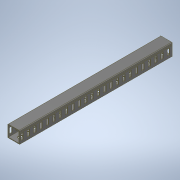
# Autodesk Inventor part: 503.009.01_Kabelkanal
Saved by Autodesk Inventor 2021 (Build 250183000, 183)
## iProperties
Created: 2021-11-27
Part Number: 503.009.01_Kabelkanal
Material: Polypropylen
Document SubType Name: Modeling
Designer: Sebastian Seewald
Density: 0.899 g/cm^3
Appearance: Glatt - Esche
Mass: 114.345 g
Surface Area: 1336.96 cm^2
Volume: 127.191 cm^3
Author: Sebastian Seewald
Autodesk Inventor part; units mm, degrees
ref_plane "YZ Plane" through (0, 0, 0) normal (1, 0, 0) x (0, 1, 0)
ref_plane "XZ Plane" through (0, 0, 0) normal (0, 1, 0) x (-1, 0, 0)
sketch "Skizze1" plane through (0, 0, 0) normal (0, 0, 1) x (1, 0, 0)
  line L0 (0, 0) -> (37.5, 0)
  line L1 (37.5, 0) -> (37.5, 35.5)
  line L2 (35.5, 37.5) -> (2, 37.5)
  line L3 (0, 35.5) -> (0, 0)
  line L4 (4, 35.5) -> (33.5, 35.5)
  line L5 (35.5, 33.5) -> (35.5, 2)
  line L6 (35.5, 2) -> (2, 2)
  line L7 (2, 2) -> (2, 33.5)
  arc A0 (2, 37.5) -> (0, 35.5) centre (2, 35.5) ccw
  arc A1 (37.5, 35.5) -> (35.5, 37.5) centre (35.5, 35.5) ccw
  arc A2 (35.5, 33.5) -> (33.5, 35.5) centre (33.5, 33.5) ccw
  arc A3 (4, 35.5) -> (2, 33.5) centre (4, 33.5) ccw
  point P0 (37.5, 37.5)
  point P1 (0, 37.5)
  dimension "d0" = 37.5
  dimension "d1" = 37.5
  dimension "d2" = 2
  dimension "d3" = 2
  dimension "d4" = 2
  dimension "d5" = 2
  dimension "d6" = 2
  constraints: 16 end point, 8 point on circle, 8 tangent, 4 centre point, 4 parallel, 4 point on line, 3 equal radius, 2 horizontal, 2 perpendicular
  measures "d0" distance of point (37.5, 37.5) point (0, 37.5)
  measures "d1" distance of L0.end point (37.5, 37.5)
  measures "d2" distance between parallel lines of L3 L7
  measures "d3" distance between parallel lines of L2 L4
  measures "d4" distance between parallel lines of L1 L5
  measures "d5" distance between parallel lines of L0 L6
  measures "d6" radius of A0
extrude "Extrusion1" add sketch "Skizze1" along normal blind 480
sketch "Skizze2" plane through (0, 0, 0) normal (-1, 0, 0) x (0, 0, 1)
  line L0 (9, 26.5) -> (15, 26.5)
  line L1 (16, 25.5) -> (16, 9)
  line L2 (15, 8) -> (9, 8)
  line L3 (8, 9) -> (8, 25.5)
  line L4 (0, 0) -> (480, 0) projected
  line L5 (0, 35.5) -> (0, 0) projected
  arc A0 (9, 26.5) -> (8, 25.5) centre (9, 25.5) ccw
  arc A1 (16, 25.5) -> (15, 26.5) centre (15, 25.5) ccw
  arc A2 (15, 8) -> (16, 9) centre (15, 9) ccw
  arc A3 (8, 9) -> (9, 8) centre (9, 9) ccw
  line L6 (29, 26.5) -> (35, 26.5)
  line L7 (36, 25.5) -> (36, 9)
  line L8 (35, 8) -> (29, 8)
  line L9 (28, 9) -> (28, 25.5)
  arc A4 (29, 26.5) -> (28, 25.5) centre (29, 25.5) ccw
  arc A5 (36, 25.5) -> (35, 26.5) centre (35, 25.5) ccw
  arc A6 (35, 8) -> (36, 9) centre (35, 9) ccw
  arc A7 (28, 9) -> (29, 8) centre (29, 9) ccw
  line L10 (49, 26.5) -> (55, 26.5)
  line L11 (56, 25.5) -> (56, 9)
  line L12 (55, 8) -> (49, 8)
  line L13 (48, 9) -> (48, 25.5)
  arc A8 (49, 26.5) -> (48, 25.5) centre (49, 25.5) ccw
  arc A9 (56, 25.5) -> (55, 26.5) centre (55, 25.5) ccw
  arc A10 (55, 8) -> (56, 9) centre (55, 9) ccw
  arc A11 (48, 9) -> (49, 8) centre (49, 9) ccw
  line L14 (69, 26.5) -> (75, 26.5)
  line L15 (76, 25.5) -> (76, 9)
  line L16 (75, 8) -> (69, 8)
  line L17 (68, 9) -> (68, 25.5)
  arc A12 (69, 26.5) -> (68, 25.5) centre (69, 25.5) ccw
  arc A13 (76, 25.5) -> (75, 26.5) centre (75, 25.5) ccw
  arc A14 (75, 8) -> (76, 9) centre (75, 9) ccw
  arc A15 (68, 9) -> (69, 8) centre (69, 9) ccw
  line L18 (89, 26.5) -> (95, 26.5)
  line L19 (96, 25.5) -> (96, 9)
  line L20 (95, 8) -> (89, 8)
  line L21 (88, 9) -> (88, 25.5)
  arc A16 (89, 26.5) -> (88, 25.5) centre (89, 25.5) ccw
  arc A17 (96, 25.5) -> (95, 26.5) centre (95, 25.5) ccw
  arc A18 (95, 8) -> (96, 9) centre (95, 9) ccw
  arc A19 (88, 9) -> (89, 8) centre (89, 9) ccw
  line L22 (109, 26.5) -> (115, 26.5)
  line L23 (116, 25.5) -> (116, 9)
  line L24 (115, 8) -> (109, 8)
  line L25 (108, 9) -> (108, 25.5)
  arc A20 (109, 26.5) -> (108, 25.5) centre (109, 25.5) ccw
  arc A21 (116, 25.5) -> (115, 26.5) centre (115, 25.5) ccw
  arc A22 (115, 8) -> (116, 9) centre (115, 9) ccw
  arc A23 (108, 9) -> (109, 8) centre (109, 9) ccw
  line L26 (129, 26.5) -> (135, 26.5)
  line L27 (136, 25.5) -> (136, 9)
  line L28 (135, 8) -> (129, 8)
  line L29 (128, 9) -> (128, 25.5)
  arc A24 (129, 26.5) -> (128, 25.5) centre (129, 25.5) ccw
  arc A25 (136, 25.5) -> (135, 26.5) centre (135, 25.5) ccw
  arc A26 (135, 8) -> (136, 9) centre (135, 9) ccw
  arc A27 (128, 9) -> (129, 8) centre (129, 9) ccw
  line L30 (149, 26.5) -> (155, 26.5)
  line L31 (156, 25.5) -> (156, 9)
  line L32 (155, 8) -> (149, 8)
  line L33 (148, 9) -> (148, 25.5)
  arc A28 (149, 26.5) -> (148, 25.5) centre (149, 25.5) ccw
  arc A29 (156, 25.5) -> (155, 26.5) centre (155, 25.5) ccw
  arc A30 (155, 8) -> (156, 9) centre (155, 9) ccw
  arc A31 (148, 9) -> (149, 8) centre (149, 9) ccw
  line L34 (169, 26.5) -> (175, 26.5)
  line L35 (176, 25.5) -> (176, 9)
  line L36 (175, 8) -> (169, 8)
  line L37 (168, 9) -> (168, 25.5)
  arc A32 (169, 26.5) -> (168, 25.5) centre (169, 25.5) ccw
  arc A33 (176, 25.5) -> (175, 26.5) centre (175, 25.5) ccw
  arc A34 (175, 8) -> (176, 9) centre (175, 9) ccw
  arc A35 (168, 9) -> (169, 8) centre (169, 9) ccw
  line L38 (189, 26.5) -> (195, 26.5)
  line L39 (196, 25.5) -> (196, 9)
  line L40 (195, 8) -> (189, 8)
  line L41 (188, 9) -> (188, 25.5)
  arc A36 (189, 26.5) -> (188, 25.5) centre (189, 25.5) ccw
  arc A37 (196, 25.5) -> (195, 26.5) centre (195, 25.5) ccw
  arc A38 (195, 8) -> (196, 9) centre (195, 9) ccw
  arc A39 (188, 9) -> (189, 8) centre (189, 9) ccw
  line L42 (209, 26.5) -> (215, 26.5)
  line L43 (216, 25.5) -> (216, 9)
  line L44 (215, 8) -> (209, 8)
  line L45 (208, 9) -> (208, 25.5)
  arc A40 (209, 26.5) -> (208, 25.5) centre (209, 25.5) ccw
  arc A41 (216, 25.5) -> (215, 26.5) centre (215, 25.5) ccw
  arc A42 (215, 8) -> (216, 9) centre (215, 9) ccw
  arc A43 (208, 9) -> (209, 8) centre (209, 9) ccw
  line L46 (229, 26.5) -> (235, 26.5)
  line L47 (236, 25.5) -> (236, 9)
  line L48 (235, 8) -> (229, 8)
  line L49 (228, 9) -> (228, 25.5)
  arc A44 (229, 26.5) -> (228, 25.5) centre (229, 25.5) ccw
  arc A45 (236, 25.5) -> (235, 26.5) centre (235, 25.5) ccw
  arc A46 (235, 8) -> (236, 9) centre (235, 9) ccw
  arc A47 (228, 9) -> (229, 8) centre (229, 9) ccw
  line L50 (249, 26.5) -> (255, 26.5)
  line L51 (256, 25.5) -> (256, 9)
  line L52 (255, 8) -> (249, 8)
  line L53 (248, 9) -> (248, 25.5)
  arc A48 (249, 26.5) -> (248, 25.5) centre (249, 25.5) ccw
  arc A49 (256, 25.5) -> (255, 26.5) centre (255, 25.5) ccw
  arc A50 (255, 8) -> (256, 9) centre (255, 9) ccw
  arc A51 (248, 9) -> (249, 8) centre (249, 9) ccw
  line L54 (269, 26.5) -> (275, 26.5)
  line L55 (276, 25.5) -> (276, 9)
  line L56 (275, 8) -> (269, 8)
  line L57 (268, 9) -> (268, 25.5)
  arc A52 (269, 26.5) -> (268, 25.5) centre (269, 25.5) ccw
  arc A53 (276, 25.5) -> (275, 26.5) centre (275, 25.5) ccw
  arc A54 (275, 8) -> (276, 9) centre (275, 9) ccw
  arc A55 (268, 9) -> (269, 8) centre (269, 9) ccw
  line L58 (289, 26.5) -> (295, 26.5)
  line L59 (296, 25.5) -> (296, 9)
  line L60 (295, 8) -> (289, 8)
  line L61 (288, 9) -> (288, 25.5)
  arc A56 (289, 26.5) -> (288, 25.5) centre (289, 25.5) ccw
  arc A57 (296, 25.5) -> (295, 26.5) centre (295, 25.5) ccw
  arc A58 (295, 8) -> (296, 9) centre (295, 9) ccw
  arc A59 (288, 9) -> (289, 8) centre (289, 9) ccw
  line L62 (309, 26.5) -> (315, 26.5)
  line L63 (316, 25.5) -> (316, 9)
  line L64 (315, 8) -> (309, 8)
  line L65 (308, 9) -> (308, 25.5)
  arc A60 (309, 26.5) -> (308, 25.5) centre (309, 25.5) ccw
  arc A61 (316, 25.5) -> (315, 26.5) centre (315, 25.5) ccw
  arc A62 (315, 8) -> (316, 9) centre (315, 9) ccw
  arc A63 (308, 9) -> (309, 8) centre (309, 9) ccw
  line L66 (329, 26.5) -> (335, 26.5)
  line L67 (336, 25.5) -> (336, 9)
  line L68 (335, 8) -> (329, 8)
  line L69 (328, 9) -> (328, 25.5)
  arc A64 (329, 26.5) -> (328, 25.5) centre (329, 25.5) ccw
  arc A65 (336, 25.5) -> (335, 26.5) centre (335, 25.5) ccw
  arc A66 (335, 8) -> (336, 9) centre (335, 9) ccw
  arc A67 (328, 9) -> (329, 8) centre (329, 9) ccw
  line L70 (349, 26.5) -> (355, 26.5)
  line L71 (356, 25.5) -> (356, 9)
  line L72 (355, 8) -> (349, 8)
  line L73 (348, 9) -> (348, 25.5)
  arc A68 (349, 26.5) -> (348, 25.5) centre (349, 25.5) ccw
  arc A69 (356, 25.5) -> (355, 26.5) centre (355, 25.5) ccw
  arc A70 (355, 8) -> (356, 9) centre (355, 9) ccw
  arc A71 (348, 9) -> (349, 8) centre (349, 9) ccw
  line L74 (369, 26.5) -> (375, 26.5)
  line L75 (376, 25.5) -> (376, 9)
  line L76 (375, 8) -> (369, 8)
  line L77 (368, 9) -> (368, 25.5)
  arc A72 (369, 26.5) -> (368, 25.5) centre (369, 25.5) ccw
  arc A73 (376, 25.5) -> (375, 26.5) centre (375, 25.5) ccw
  arc A74 (375, 8) -> (376, 9) centre (375, 9) ccw
  arc A75 (368, 9) -> (369, 8) centre (369, 9) ccw
  line L78 (389, 26.5) -> (395, 26.5)
  line L79 (396, 25.5) -> (396, 9)
  line L80 (395, 8) -> (389, 8)
  line L81 (388, 9) -> (388, 25.5)
  arc A76 (389, 26.5) -> (388, 25.5) centre (389, 25.5) ccw
  arc A77 (396, 25.5) -> (395, 26.5) centre (395, 25.5) ccw
  arc A78 (395, 8) -> (396, 9) centre (395, 9) ccw
  arc A79 (388, 9) -> (389, 8) centre (389, 9) ccw
  line L82 (409, 26.5) -> (415, 26.5)
  line L83 (416, 25.5) -> (416, 9)
  line L84 (415, 8) -> (409, 8)
  line L85 (408, 9) -> (408, 25.5)
  arc A80 (409, 26.5) -> (408, 25.5) centre (409, 25.5) ccw
  arc A81 (416, 25.5) -> (415, 26.5) centre (415, 25.5) ccw
  arc A82 (415, 8) -> (416, 9) centre (415, 9) ccw
  arc A83 (408, 9) -> (409, 8) centre (409, 9) ccw
  line L86 (429, 26.5) -> (435, 26.5)
  line L87 (436, 25.5) -> (436, 9)
  line L88 (435, 8) -> (429, 8)
  line L89 (428, 9) -> (428, 25.5)
  arc A84 (429, 26.5) -> (428, 25.5) centre (429, 25.5) ccw
  arc A85 (436, 25.5) -> (435, 26.5) centre (435, 25.5) ccw
  arc A86 (435, 8) -> (436, 9) centre (435, 9) ccw
  arc A87 (428, 9) -> (429, 8) centre (429, 9) ccw
  line L90 (449, 26.5) -> (455, 26.5)
  line L91 (456, 25.5) -> (456, 9)
  line L92 (455, 8) -> (449, 8)
  line L93 (448, 9) -> (448, 25.5)
  arc A88 (449, 26.5) -> (448, 25.5) centre (449, 25.5) ccw
  arc A89 (456, 25.5) -> (455, 26.5) centre (455, 25.5) ccw
  arc A90 (455, 8) -> (456, 9) centre (455, 9) ccw
  arc A91 (448, 9) -> (449, 8) centre (449, 9) ccw
  line L94 (469, 26.5) -> (475, 26.5)
  line L95 (476, 25.5) -> (476, 9)
  line L96 (475, 8) -> (469, 8)
  line L97 (468, 9) -> (468, 25.5)
  arc A92 (469, 26.5) -> (468, 25.5) centre (469, 25.5) ccw
  arc A93 (476, 25.5) -> (475, 26.5) centre (475, 25.5) ccw
  arc A94 (475, 8) -> (476, 9) centre (475, 9) ccw
  arc A95 (468, 9) -> (469, 8) centre (469, 9) ccw
  line L98 (489, 26.5) -> (495, 26.5)
  line L99 (496, 25.5) -> (496, 9)
  line L100 (495, 8) -> (489, 8)
  line L101 (488, 9) -> (488, 25.5)
  arc A96 (489, 26.5) -> (488, 25.5) centre (489, 25.5) ccw
  arc A97 (496, 25.5) -> (495, 26.5) centre (495, 25.5) ccw
  arc A98 (495, 8) -> (496, 9) centre (495, 9) ccw
  arc A99 (488, 9) -> (489, 8) centre (489, 9) ccw
  dimension "d11" = 8
  dimension "d12" = 8
  dimension "d13" = 8
  dimension "d14" = 18.5
  dimension "d15" = 1
  dimension "d18" = 20
  constraints: 200 end point, 200 point on circle, 100 centre point, 8 tangent, 3 equal radius, 2 horizontal, 2 parallel, 1 perpendicular, 480 other
  measures "d11" distance between parallel lines of L4 L2
  measures "d12" distance between parallel lines of L3 L1
  measures "d13" distance between parallel lines of L5 L3
  measures "d14" distance between parallel lines of L2 L0
  measures "d15" radius of A0
  measures "d18" distance of L0.start L6.start
extrude "Extrusion2" cut sketch "Skizze2" against normal up to surface (37.5 mm away)
sketch "Skizze3" plane through (0, 0, 0) normal (0, -1, 0) x (1, 0, 0)
  line L0 (18.75, 463.75) -> (18.75, 456.25) construction
  line L1 (15.5, 463.75) -> (15.5, 456.25)
  line L2 (22, 456.25) -> (22, 463.75)
  arc A0 (22, 463.75) -> (15.5, 463.75) centre (18.75, 463.75) ccw
  arc A1 (15.5, 456.25) -> (22, 456.25) centre (18.75, 456.25) ccw
  line L3 (18.75, 436.75) -> (18.75, 433.25) construction
  line L4 (16.5, 436.75) -> (16.5, 433.25)
  line L5 (21, 433.25) -> (21, 436.75)
  arc A2 (21, 436.75) -> (16.5, 436.75) centre (18.75, 436.75) ccw
  arc A3 (16.5, 433.25) -> (21, 433.25) centre (18.75, 433.25) ccw
  line L6 (0, 480) -> (37.5, 480) projected
  line L7 (37.5, 0) -> (37.5, 480) projected
  arc A4 (15.5, 406.25) -> (22, 406.25) centre (18.75, 406.25) ccw
  line L8 (18.75, 413.75) -> (18.75, 406.25) construction
  line L9 (22, 406.25) -> (22, 413.75)
  line L10 (15.5, 413.75) -> (15.5, 406.25)
  arc A5 (22, 413.75) -> (15.5, 413.75) centre (18.75, 413.75) ccw
  arc A6 (21, 386.75) -> (16.5, 386.75) centre (18.75, 386.75) ccw
  line L11 (16.5, 386.75) -> (16.5, 383.25)
  line L12 (21, 383.25) -> (21, 386.75)
  arc A7 (16.5, 383.25) -> (21, 383.25) centre (18.75, 383.25) ccw
  arc A8 (15.5, 356.25) -> (22, 356.25) centre (18.75, 356.25) ccw
  line L13 (18.75, 363.75) -> (18.75, 356.25) construction
  line L14 (22, 356.25) -> (22, 363.75)
  line L15 (15.5, 363.75) -> (15.5, 356.25)
  arc A9 (22, 363.75) -> (15.5, 363.75) centre (18.75, 363.75) ccw
  arc A10 (21, 336.75) -> (16.5, 336.75) centre (18.75, 336.75) ccw
  line L16 (16.5, 336.75) -> (16.5, 333.25)
  line L17 (21, 333.25) -> (21, 336.75)
  arc A11 (16.5, 333.25) -> (21, 333.25) centre (18.75, 333.25) ccw
  arc A12 (15.5, 306.25) -> (22, 306.25) centre (18.75, 306.25) ccw
  line L18 (18.75, 313.75) -> (18.75, 306.25) construction
  line L19 (22, 306.25) -> (22, 313.75)
  line L20 (15.5, 313.75) -> (15.5, 306.25)
  arc A13 (22, 313.75) -> (15.5, 313.75) centre (18.75, 313.75) ccw
  arc A14 (21, 286.75) -> (16.5, 286.75) centre (18.75, 286.75) ccw
  line L21 (16.5, 286.75) -> (16.5, 283.25)
  line L22 (21, 283.25) -> (21, 286.75)
  arc A15 (16.5, 283.25) -> (21, 283.25) centre (18.75, 283.25) ccw
  arc A16 (15.5, 256.25) -> (22, 256.25) centre (18.75, 256.25) ccw
  line L23 (18.75, 263.75) -> (18.75, 256.25) construction
  line L24 (22, 256.25) -> (22, 263.75)
  line L25 (15.5, 263.75) -> (15.5, 256.25)
  arc A17 (22, 263.75) -> (15.5, 263.75) centre (18.75, 263.75) ccw
  arc A18 (21, 236.75) -> (16.5, 236.75) centre (18.75, 236.75) ccw
  line L26 (16.5, 236.75) -> (16.5, 233.25)
  line L27 (21, 233.25) -> (21, 236.75)
  arc A19 (16.5, 233.25) -> (21, 233.25) centre (18.75, 233.25) ccw
  arc A20 (15.5, 206.25) -> (22, 206.25) centre (18.75, 206.25) ccw
  line L28 (18.75, 213.75) -> (18.75, 206.25) construction
  line L29 (22, 206.25) -> (22, 213.75)
  line L30 (15.5, 213.75) -> (15.5, 206.25)
  arc A21 (22, 213.75) -> (15.5, 213.75) centre (18.75, 213.75) ccw
  arc A22 (21, 186.75) -> (16.5, 186.75) centre (18.75, 186.75) ccw
  line L31 (16.5, 186.75) -> (16.5, 183.25)
  line L32 (21, 183.25) -> (21, 186.75)
  arc A23 (16.5, 183.25) -> (21, 183.25) centre (18.75, 183.25) ccw
  arc A24 (15.5, 156.25) -> (22, 156.25) centre (18.75, 156.25) ccw
  line L33 (18.75, 163.75) -> (18.75, 156.25) construction
  line L34 (22, 156.25) -> (22, 163.75)
  line L35 (15.5, 163.75) -> (15.5, 156.25)
  arc A25 (22, 163.75) -> (15.5, 163.75) centre (18.75, 163.75) ccw
  arc A26 (21, 136.75) -> (16.5, 136.75) centre (18.75, 136.75) ccw
  line L36 (16.5, 136.75) -> (16.5, 133.25)
  line L37 (21, 133.25) -> (21, 136.75)
  arc A27 (16.5, 133.25) -> (21, 133.25) centre (18.75, 133.25) ccw
  arc A28 (15.5, 106.25) -> (22, 106.25) centre (18.75, 106.25) ccw
  line L38 (18.75, 113.75) -> (18.75, 106.25) construction
  line L39 (22, 106.25) -> (22, 113.75)
  line L40 (15.5, 113.75) -> (15.5, 106.25)
  arc A29 (22, 113.75) -> (15.5, 113.75) centre (18.75, 113.75) ccw
  arc A30 (21, 86.75) -> (16.5, 86.75) centre (18.75, 86.75) ccw
  line L41 (16.5, 86.75) -> (16.5, 83.25)
  line L42 (21, 83.25) -> (21, 86.75)
  arc A31 (16.5, 83.25) -> (21, 83.25) centre (18.75, 83.25) ccw
  arc A32 (15.5, 56.25) -> (22, 56.25) centre (18.75, 56.25) ccw
  line L43 (18.75, 63.75) -> (18.75, 56.25) construction
  line L44 (22, 56.25) -> (22, 63.75)
  line L45 (15.5, 63.75) -> (15.5, 56.25)
  arc A33 (22, 63.75) -> (15.5, 63.75) centre (18.75, 63.75) ccw
  arc A34 (21, 36.75) -> (16.5, 36.75) centre (18.75, 36.75) ccw
  line L46 (16.5, 36.75) -> (16.5, 33.25)
  line L47 (21, 33.25) -> (21, 36.75)
  arc A35 (16.5, 33.25) -> (21, 33.25) centre (18.75, 33.25) ccw
  arc A36 (15.5, 6.25) -> (22, 6.25) centre (18.75, 6.25) ccw
  line L48 (18.75, 13.75) -> (18.75, 6.25) construction
  line L49 (22, 6.25) -> (22, 13.75)
  line L50 (15.5, 13.75) -> (15.5, 6.25)
  arc A37 (22, 13.75) -> (15.5, 13.75) centre (18.75, 13.75) ccw
  arc A38 (21, -13.25) -> (16.5, -13.25) centre (18.75, -13.25) ccw
  line L51 (16.5, -13.25) -> (16.5, -16.75)
  line L52 (21, -16.75) -> (21, -13.25)
  arc A39 (16.5, -16.75) -> (21, -16.75) centre (18.75, -16.75) ccw
  point P0 (0, 0)
  point P1 (18.75, 460)
  point P2 (18.75, 435)
  point P3 (18.75, 410)
  point P4 (18.75, 385)
  point P5 (18.75, 360)
  point P6 (18.75, 335)
  point P7 (18.75, 310)
  point P8 (18.75, 285)
  point P9 (18.75, 260)
  point P10 (18.75, 235)
  point P11 (18.75, 210)
  point P12 (18.75, 185)
  point P13 (18.75, 160)
  point P14 (18.75, 135)
  point P15 (18.75, 110)
  point P16 (18.75, 85)
  point P17 (18.75, 60)
  point P18 (18.75, 35)
  point P19 (18.75, 10)
  point P20 (18.75, -15)
  dimension "d25" = 7.5
  dimension "d26" = 6.5
  dimension "d27" = 3.5
  dimension "d28" = 4.5
  dimension "d29" = 25
  dimension "d30" = 20
  dimension "d31" = 18.75
  dimension "d34" = 50
  constraints: 124 end point, 80 point on circle, 40 centre point, 20 point on line, 8 tangent, 2 midpoint, 2 parallel, 2 vertical, 207 other
  measures "d25" distance of L0.start L0.end
  measures "d26" distance between parallel lines of L1 L2
  measures "d27" distance of L3.start L3.end
  measures "d28" distance between parallel lines of L4 L5
  measures "d29" distance of point (18.75, 435) point (18.75, 460)
  measures "d30" distance from line of L6 point (18.75, 460)
  measures "d31" distance between parallel lines of L7 L0
  measures "d34" distance of L1.end L10.end
extrude "Extrusion3" cut sketch "Skizze3" against normal up to surface (2 mm away)
sketch "Skizze4" plane through (0, 0, 480) normal (0, 0, 1) x (1, 0, 0)
  line L0 (0, 35.5) -> (0, 0) projected
  line L1 (0, 31.5) -> (0.6498, 31.5)
  line L2 (0.6498, 31.5) -> (0, 29.5)
  line L3 (0, 29.5) -> (0, 31.5)
  line L4 (2, 2) -> (2, 33.5) projected
  line L5 (35.5, 37.5) -> (2, 37.5) projected
  dimension "d41" = 18
  dimension "d42" = 8
  dimension "d43" = 90
  dimension "d44" = 2
  constraints: 6 end point, 1 point on line, 1 vertical
  measures "d41" angle of L4 L2
  measures "d42" distance from line of L5 L2.end
  measures "d43" angle of L0 L1
  measures "d44" distance from line of L2.end L1
extrude "Extrusion4" cut sketch "Skizze4" against normal up to surface (480 mm away)
ref_plane "Arbeitsebene1" through (18.75, 0, 0) normal (-1, 0, 0) x (0, 0, 1)
mirror "Spiegeln1" about plane through (18.75, 0, 0) normal (-1, 0, 0) of "Extrusion4"
